Autodesk Inventor part; units mm, degrees
(part 2 of 3)
  spline S187 degree 2 poles (-30.3145, -0.1752) (-30.3145, 0.4002) (-30.6954, 1.2146) (-31.0722, 1.4456) knots 0 0 0 1 2 2 2
  spline S188 degree 2 poles (-31.0722, 1.4456) (-31.3396, 1.6036) (-31.9433, 1.7454) (-32.3931, 1.7454) knots 0 0 0 1 2 2 2
  line L488 (-32.3931, 1.7454) -> (-32.8996, 1.7454)
  line L489 (-32.8996, 1.7454) -> (-32.8996, -2.1038)
  line L490 (-32.8996, -2.1038) -> (-32.3931, -2.1038)
  spline S189 degree 2 poles (-32.3931, -2.1038) (-31.9514, -2.1038) (-31.2829, -1.962) (-31.0114, -1.7716) knots 0 0 0 1 2 2 2
  spline S190 degree 2 poles (-31.0114, -1.7716) (-30.6629, -1.5366) (-30.3145, -0.7586) (-30.3145, -0.1752) knots 0 0 0 1 2 2 2
  line L491 (-23.1062, -2.6792) -> (-23.9693, -2.6792)
  line L492 (-23.9693, -2.6792) -> (-25.7967, -0.3534)
  line L493 (-25.7967, -0.3534) -> (-26.0884, -0.6816)
  line L494 (-26.0884, -0.6816) -> (-26.0884, -2.6792)
  line L495 (-26.0884, -2.6792) -> (-26.7529, -2.6792)
  line L496 (-26.7529, -2.6792) -> (-26.7529, 2.3208)
  line L497 (-26.7529, 2.3208) -> (-26.0884, 2.3208)
  line L498 (-26.0884, 2.3208) -> (-26.0884, 0.0234)
  line L499 (-26.0884, 0.0234) -> (-24.0381, 2.3208)
  line L500 (-24.0381, 2.3208) -> (-23.2278, 2.3208)
  line L501 (-23.2278, 2.3208) -> (-25.2983, 0.0882)
  line L502 (-25.2983, 0.0882) -> (-23.1062, -2.6792)
  line L503 (-20.9668, -2.6792) -> (-22.9036, -2.6792)
  line L504 (-22.9036, -2.6792) -> (-22.9036, -2.1687)
  line L505 (-22.9036, -2.1687) -> (-22.2675, -2.1687)
  line L506 (-22.2675, -2.1687) -> (-22.2675, 1.8103)
  line L507 (-22.2675, 1.8103) -> (-22.9036, 1.8103)
  line L508 (-22.9036, 1.8103) -> (-22.9036, 2.3208)
  line L509 (-22.9036, 2.3208) -> (-20.9668, 2.3208)
  line L510 (-20.9668, 2.3208) -> (-20.9668, 1.8103)
  line L511 (-20.9668, 1.8103) -> (-21.603, 1.8103)
  line L512 (-21.603, 1.8103) -> (-21.603, -2.1687)
  line L513 (-21.603, -2.1687) -> (-20.9668, -2.1687)
  line L514 (-20.9668, -2.1687) -> (-20.9668, -2.6792)
  line L515 (-20.1443, -2.6792) -> (-20.1443, 2.3208)
  line L516 (-20.1443, 2.3208) -> (-17.0163, 2.3208)
  line L517 (-17.0163, 2.3208) -> (-17.0163, 1.7292)
  line L518 (-17.0163, 1.7292) -> (-19.4798, 1.7292)
  line L519 (-19.4798, 1.7292) -> (-19.4798, 0.3597)
  line L520 (-19.4798, 0.3597) -> (-17.1824, 0.3597)
  line L521 (-17.1824, 0.3597) -> (-17.1824, -0.2319)
  line L522 (-17.1824, -0.2319) -> (-19.4798, -0.2319)
  line L523 (-19.4798, -0.2319) -> (-19.4798, -2.0876)
  line L524 (-19.4798, -2.0876) -> (-17.0163, -2.0876)
  line L525 (-17.0163, -2.0876) -> (-17.0163, -2.6792)
  line L526 (-17.0163, -2.6792) -> (-20.1443, -2.6792)
  line L527 (-12.4174, -2.6792) -> (-13.2804, -2.6792)
  line L528 (-13.2804, -2.6792) -> (-14.8607, -0.6897)
  line L529 (-14.8607, -0.6897) -> (-15.6224, -0.6897)
  line L530 (-15.6224, -0.6897) -> (-15.6224, -2.6792)
  line L531 (-15.6224, -2.6792) -> (-16.2869, -2.6792)
  line L532 (-16.2869, -2.6792) -> (-16.2869, 2.3208)
  line L533 (-16.2869, 2.3208) -> (-14.9984, 2.3208)
  spline S191 degree 2 poles (-14.9984, 2.3208) (-14.5689, 2.3208) (-13.9895, 2.2276) (-13.7262, 2.0574) knots 0 0 0 1 2 2 2
  spline S192 degree 2 poles (-13.7262, 2.0574) (-13.4628, 1.8872) (-13.1589, 1.3564) (-13.1589, 0.9634) knots 0 0 0 1 2 2 2
  spline S193 degree 2 poles (-13.1589, 0.9634) (-13.1589, 0.4164) (-13.7181, -0.3251) (-14.1962, -0.5034) knots 0 0 0 1 2 2 2
  line L534 (-14.1962, -0.5034) -> (-12.4174, -2.6792)
  spline S194 degree 2 poles (-13.8518, 0.9107) (-13.8518, 1.1295) (-14.0057, 1.4658) (-14.1678, 1.5752) knots 0 0 0 1 2 2 2
  spline S195 degree 2 poles (-14.1678, 1.5752) (-14.3096, 1.6684) (-14.6864, 1.7454) (-14.962, 1.7454) knots 0 0 0 1 2 2 2
  line L535 (-14.962, 1.7454) -> (-15.6224, 1.7454)
  line L536 (-15.6224, 1.7454) -> (-15.6224, -0.1346)
  line L537 (-15.6224, -0.1346) -> (-15.039, -0.1346)
  spline S196 degree 2 poles (-15.039, -0.1346) (-14.7513, -0.1346) (-14.2934, -0.0333) (-14.1354, 0.1247) knots 0 0 0 1 2 2 2
  spline S197 degree 2 poles (-14.1354, 0.1247) (-13.9895, 0.2624) (-13.8518, 0.6514) (-13.8518, 0.9107) knots 0 0 0 1 2 2 2
  spline S198 degree 2 poles (-10.274, -2.7846) (-10.7156, -2.7846) (-11.372, -2.5536) (-11.603, -2.3226) knots 0 0 0 1 2 2 2
  spline S199 degree 2 poles (-11.603, -2.3226) (-11.8663, -2.0633) (-12.0811, -1.334) (-12.0811, -0.7991) knots 0 0 0 1 2 2 2
  line L538 (-12.0811, -0.7991) -> (-12.0811, 2.3208)
  line L539 (-12.0811, 2.3208) -> (-11.4166, 2.3208)
  line L540 (-11.4166, 2.3208) -> (-11.4166, -0.7991)
  spline S200 degree 2 poles (-11.4166, -0.7991) (-11.4166, -1.1476) (-11.3275, -1.6176) (-11.2018, -1.8081) knots 0 0 0 1 2 2 2
  spline S201 degree 2 poles (-11.2018, -1.8081) (-11.0681, -2.0107) (-10.6062, -2.2173) (-10.274, -2.2173) knots 0 0 0 1 2 2 2
  spline S202 degree 2 poles (-10.274, -2.2173) (-9.962, -2.2173) (-9.4757, -2.0107) (-9.342, -1.8081) knots 0 0 0 1 2 2 2
  spline S203 degree 2 poles (-9.342, -1.8081) (-9.2164, -1.6176) (-9.1273, -1.1517) (-9.1273, -0.8154) knots 0 0 0 1 2 2 2
  line L541 (-9.1273, -0.8154) -> (-9.1273, 2.3208)
  line L542 (-9.1273, 2.3208) -> (-8.4628, 2.3208)
  line L543 (-8.4628, 2.3208) -> (-8.4628, -0.7991)
  spline S204 degree 2 poles (-8.4628, -0.7991) (-8.4628, -1.3218) (-8.6735, -2.0674) (-8.9409, -2.3226) knots 0 0 0 1 2 2 2
  spline S205 degree 2 poles (-8.9409, -2.3226) (-9.18, -2.5577) (-9.8121, -2.7846) (-10.274, -2.7846) knots 0 0 0 1 2 2 2
  line L544 (-3.9328, -2.6792) -> (-4.6783, -2.6792)
  line L545 (-4.6783, -2.6792) -> (-6.8907, 1.632)
  line L546 (-6.8907, 1.632) -> (-6.8907, -2.6792)
  line L547 (-6.8907, -2.6792) -> (-7.5106, -2.6792)
  line L548 (-7.5106, -2.6792) -> (-7.5106, 2.3208)
  line L549 (-7.5106, 2.3208) -> (-6.5665, 2.3208)
  line L550 (-6.5665, 2.3208) -> (-4.5527, -1.6379)
  line L551 (-4.5527, -1.6379) -> (-4.5527, 2.3208)
  line L552 (-4.5527, 2.3208) -> (-3.9328, 2.3208)
  line L553 (-3.9328, 2.3208) -> (-3.9328, -2.6792)
  line L554 (0.7268, -2.6792) -> (-0.1362, -2.6792)
  line L555 (-0.1362, -2.6792) -> (-1.9636, -0.3534)
  line L556 (-1.9636, -0.3534) -> (-2.2553, -0.6816)
  line L557 (-2.2553, -0.6816) -> (-2.2553, -2.6792)
  line L558 (-2.2553, -2.6792) -> (-2.9198, -2.6792)
  line L559 (-2.9198, -2.6792) -> (-2.9198, 2.3208)
  line L560 (-2.9198, 2.3208) -> (-2.2553, 2.3208)
  line L561 (-2.2553, 2.3208) -> (-2.2553, 0.0234)
  line L562 (-2.2553, 0.0234) -> (-0.2051, 2.3208)
  line L563 (-0.2051, 2.3208) -> (0.6053, 2.3208)
  line L564 (0.6053, 2.3208) -> (-1.4652, 0.0882)
  line L565 (-1.4652, 0.0882) -> (0.7268, -2.6792)
  line L566 (2.8662, -2.6792) -> (0.9294, -2.6792)
  line L567 (0.9294, -2.6792) -> (0.9294, -2.1687)
  line L568 (0.9294, -2.1687) -> (1.5656, -2.1687)
  line L569 (1.5656, -2.1687) -> (1.5656, 1.8103)
  line L570 (1.5656, 1.8103) -> (0.9294, 1.8103)
  line L571 (0.9294, 1.8103) -> (0.9294, 2.3208)
  line L572 (0.9294, 2.3208) -> (2.8662, 2.3208)
  line L573 (2.8662, 2.3208) -> (2.8662, 1.8103)
  line L574 (2.8662, 1.8103) -> (2.2301, 1.8103)
  line L575 (2.2301, 1.8103) -> (2.2301, -2.1687)
  line L576 (2.2301, -2.1687) -> (2.8662, -2.1687)
  line L577 (2.8662, -2.1687) -> (2.8662, -2.6792)
  line L578 (3.6888, -2.6792) -> (3.6888, 2.3208)
  line L579 (3.6888, 2.3208) -> (6.8168, 2.3208)
  line L580 (6.8168, 2.3208) -> (6.8168, 1.7292)
  line L581 (6.8168, 1.7292) -> (4.3533, 1.7292)
  line L582 (4.3533, 1.7292) -> (4.3533, 0.3597)
  line L583 (4.3533, 0.3597) -> (6.6507, 0.3597)
  line L584 (6.6507, 0.3597) -> (6.6507, -0.2319)
  line L585 (6.6507, -0.2319) -> (4.3533, -0.2319)
  line L586 (4.3533, -0.2319) -> (4.3533, -2.0876)
  line L587 (4.3533, -2.0876) -> (6.8168, -2.0876)
  line L588 (6.8168, -2.0876) -> (6.8168, -2.6792)
  line L589 (6.8168, -2.6792) -> (3.6888, -2.6792)
  line L590 (11.833, -2.6792) -> (11.1685, -2.6792)
  line L591 (11.1685, -2.6792) -> (11.1685, 1.6279)
  line L592 (11.1685, 1.6279) -> (9.8638, -1.3016)
  line L593 (9.8638, -1.3016) -> (9.4586, -1.3016)
  line L594 (9.4586, -1.3016) -> (8.1661, 1.6279)
  line L595 (8.1661, 1.6279) -> (8.1661, -2.6792)
  line L596 (8.1661, -2.6792) -> (7.5461, -2.6792)
  line L597 (7.5461, -2.6792) -> (7.5461, 2.3208)
  line L598 (7.5461, 2.3208) -> (8.4537, 2.3208)
  line L599 (8.4537, 2.3208) -> (9.7017, -0.4628)
  line L600 (9.7017, -0.4628) -> (10.9092, 2.3208)
  line L601 (10.9092, 2.3208) -> (11.833, 2.3208)
  line L602 (11.833, 2.3208) -> (11.833, -2.6792)
  line L603 (16.7358, -2.6792) -> (14.799, -2.6792)
  line L604 (14.799, -2.6792) -> (14.799, -2.1687)
  line L605 (14.799, -2.1687) -> (15.4351, -2.1687)
  line L606 (15.4351, -2.1687) -> (15.4351, 1.8103)
  line L607 (15.4351, 1.8103) -> (14.799, 1.8103)
  line L608 (14.799, 1.8103) -> (14.799, 2.3208)
  line L609 (14.799, 2.3208) -> (16.7358, 2.3208)
  line L610 (16.7358, 2.3208) -> (16.7358, 1.8103)
  line L611 (16.7358, 1.8103) -> (16.0996, 1.8103)
  line L612 (16.0996, 1.8103) -> (16.0996, -2.1687)
  line L613 (16.0996, -2.1687) -> (16.7358, -2.1687)
  line L614 (16.7358, -2.1687) -> (16.7358, -2.6792)
  spline S206 degree 2 poles (23.2431, 1.7495) (23.5267, 1.4172) (23.8427, 0.4448) (23.8427, -0.1792) knots 0 0 0 1 2 2 2
  spline S207 degree 2 poles (23.8427, -0.1792) (23.8427, -0.787) (23.5348, -1.7716) (23.2431, -2.1038) knots 0 0 0 1 2 2 2
  spline S208 degree 2 poles (23.2431, -2.1038) (22.9351, -2.4523) (22.1207, -2.7846) (21.6304, -2.7846) knots 0 0 0 1 2 2 2
  spline S209 degree 2 poles (21.6304, -2.7846) (21.1239, -2.7846) (20.3136, -2.4402) (20.0178, -2.1038) knots 0 0 0 1 2 2 2
  spline S210 degree 2 poles (20.0178, -2.1038) (19.7301, -1.7716) (19.4221, -0.7951) (19.4221, -0.1792) knots 0 0 0 1 2 2 2
  spline S211 degree 2 poles (19.4221, -0.1792) (19.4221, 0.4488) (19.7341, 1.4051) (20.0218, 1.7495) knots 0 0 0 1 2 2 2
  spline S212 degree 2 poles (20.0218, 1.7495) (20.3136, 2.0817) (21.128, 2.4261) (21.6304, 2.4261) knots 0 0 0 1 2 2 2
  spline S213 degree 2 poles (21.6304, 2.4261) (22.1409, 2.4261) (22.9594, 2.0696) (23.2431, 1.7495) knots 0 0 0 1 2 2 2
  spline S214 degree 2 poles (23.1499, -0.1792) (23.1499, 0.3151) (22.9351, 1.0809) (22.7406, 1.3321) knots 0 0 0 1 2 2 2
  spline S215 degree 2 poles (22.7406, 1.3321) (22.5421, 1.5915) (21.9829, 1.8508) (21.6345, 1.8508) knots 0 0 0 1 2 2 2
  spline S216 degree 2 poles (21.6345, 1.8508) (21.2738, 1.8508) (20.7309, 1.5996) (20.5243, 1.3321) knots 0 0 0 1 2 2 2
  spline S217 degree 2 poles (20.5243, 1.3321) (20.3257, 1.0769) (20.115, 0.307) (20.115, -0.1792) knots 0 0 0 1 2 2 2
  spline S218 degree 2 poles (20.115, -0.1792) (20.115, -1.1638) (20.9416, -2.2092) (21.6345, -2.2092) knots 0 0 0 1 2 2 2
  spline S219 degree 2 poles (21.6345, -2.2092) (22.3273, -2.2092) (23.1499, -1.1638) (23.1499, -0.1792) knots 0 0 0 1 2 2 2
  spline S220 degree 2 poles (27.7325, 0.8135) (27.7325, 0.4893) (27.5016, -0.0941) (27.2949, -0.2967) knots 0 0 0 1 2 2 2
  spline S221 degree 2 poles (27.2949, -0.2967) (27.0356, -0.552) (26.3346, -0.8154) (25.7998, -0.8154) knots 0 0 0 1 2 2 2
  line L615 (25.7998, -0.8154) -> (25.2366, -0.8154)
  line L616 (25.2366, -0.8154) -> (25.2366, -2.6792)
  line L617 (25.2366, -2.6792) -> (24.5721, -2.6792)
  line L618 (24.5721, -2.6792) -> (24.5721, 2.3208)
  line L619 (24.5721, 2.3208) -> (25.8281, 2.3208)
  spline S222 degree 2 poles (25.8281, 2.3208) (26.2738, 2.3208) (26.8978, 2.1749) (27.1369, 2.0088) knots 0 0 0 1 2 2 2
  spline S223 degree 2 poles (27.1369, 2.0088) (27.4165, 1.8184) (27.7325, 1.2308) (27.7325, 0.8135) knots 0 0 0 1 2 2 2
  spline S224 degree 2 poles (27.0396, 0.7932) (27.0396, 1.0526) (26.8614, 1.4334) (26.679, 1.555) knots 0 0 0 1 2 2 2
  spline S225 degree 2 poles (26.679, 1.555) (26.521, 1.6603) (26.0996, 1.7454) (25.7876, 1.7454) knots 0 0 0 1 2 2 2
  line L620 (25.7876, 1.7454) -> (25.2366, 1.7454)
  line L621 (25.2366, 1.7454) -> (25.2366, -0.2481)
  line L622 (25.2366, -0.2481) -> (25.6904, -0.2481)
  spline S226 degree 2 poles (25.6904, -0.2481) (26.0956, -0.2481) (26.5939, -0.1184) (26.756, 0.0517) knots 0 0 0 1 2 2 2
  spline S227 degree 2 poles (26.756, 0.0517) (26.9059, 0.2017) (27.0396, 0.5542) (27.0396, 0.7932) knots 0 0 0 1 2 2 2
  line L623 (30.1069, -2.6792) -> (28.1701, -2.6792)
  line L624 (28.1701, -2.6792) -> (28.1701, -2.1687)
  line L625 (28.1701, -2.1687) -> (28.8063, -2.1687)
  line L626 (28.8063, -2.1687) -> (28.8063, 1.8103)
  line L627 (28.8063, 1.8103) -> (28.1701, 1.8103)
  line L628 (28.1701, 1.8103) -> (28.1701, 2.3208)
  line L629 (28.1701, 2.3208) -> (30.1069, 2.3208)
  line L630 (30.1069, 2.3208) -> (30.1069, 1.8103)
  line L631 (30.1069, 1.8103) -> (29.4708, 1.8103)
  line L632 (29.4708, 1.8103) -> (29.4708, -2.1687)
  line L633 (29.4708, -2.1687) -> (30.1069, -2.1687)
  line L634 (30.1069, -2.1687) -> (30.1069, -2.6792)
  line L635 (30.9294, -2.6792) -> (30.9294, 2.3208)
  line L636 (30.9294, 2.3208) -> (34.0575, 2.3208)
  line L637 (34.0575, 2.3208) -> (34.0575, 1.7292)
  line L638 (34.0575, 1.7292) -> (31.5939, 1.7292)
  line L639 (31.5939, 1.7292) -> (31.5939, 0.3597)
  line L640 (31.5939, 0.3597) -> (33.8913, 0.3597)
  line L641 (33.8913, 0.3597) -> (33.8913, -0.2319)
  line L642 (33.8913, -0.2319) -> (31.5939, -0.2319)
  line L643 (31.5939, -0.2319) -> (31.5939, -2.0876)
  line L644 (31.5939, -2.0876) -> (34.0575, -2.0876)
  line L645 (34.0575, -2.0876) -> (34.0575, -2.6792)
  line L646 (34.0575, -2.6792) -> (30.9294, -2.6792)
  line L647 (38.4335, -2.6792) -> (37.5704, -2.6792)
  line L648 (37.5704, -2.6792) -> (35.7431, -0.3534)
  line L649 (35.7431, -0.3534) -> (35.4513, -0.6816)
  line L650 (35.4513, -0.6816) -> (35.4513, -2.6792)
  line L651 (35.4513, -2.6792) -> (34.7868, -2.6792)
  line L652 (34.7868, -2.6792) -> (34.7868, 2.3208)
  line L653 (34.7868, 2.3208) -> (35.4513, 2.3208)
  line L654 (35.4513, 2.3208) -> (35.4513, 0.0234)
  line L655 (35.4513, 0.0234) -> (37.5016, 2.3208)
  line L656 (37.5016, 2.3208) -> (38.3119, 2.3208)
  line L657 (38.3119, 2.3208) -> (36.2414, 0.0882)
  line L658 (36.2414, 0.0882) -> (38.4335, -2.6792)
  line L659 (38.2917, -2.6792) -> (39.9772, 2.3208)
  line L660 (39.9772, 2.3208) -> (40.7957, 2.3208)
  line L661 (40.7957, 2.3208) -> (42.4813, -2.6792)
  line L662 (42.4813, -2.6792) -> (41.7803, -2.6792)
  line L663 (41.7803, -2.6792) -> (41.3265, -1.2813)
  line L664 (41.3265, -1.2813) -> (39.4181, -1.2813)
  line L665 (39.4181, -1.2813) -> (38.9643, -2.6792)
  line L666 (38.9643, -2.6792) -> (38.2917, -2.6792)
  line L667 (41.1442, -0.7141) -> (40.3703, 1.6401)
  line L668 (40.3703, 1.6401) -> (39.6004, -0.7141)
  line L669 (39.6004, -0.7141) -> (41.1442, -0.7141)
  spline S228 degree 2 poles (42.3597, -2.6792) (42.2139, -2.8008) (41.9951, -3.1614) (41.9951, -3.3194) knots 0 0 0 1 2 2 2
  spline S229 degree 2 poles (41.9951, -3.3194) (41.9951, -3.4288) (42.1207, -3.5666) (42.2463, -3.5666) knots 0 0 0 1 2 2 2
  spline S230 degree 2 poles (42.2463, -3.5666) (42.3152, -3.5666) (42.4408, -3.5342) (42.4813, -3.5179) knots 0 0 0 1 2 2 2
  line L670 (42.4813, -3.5179) -> (42.5178, -3.5179)
  line L671 (42.5178, -3.5179) -> (42.5178, -3.988)
  spline S231 degree 2 poles (42.5178, -3.988) (42.4205, -4.0285) (42.2058, -4.065) (42.1166, -4.065) knots 0 0 0 1 2 2 2
  spline S232 degree 2 poles (42.1166, -4.065) (41.8168, -4.065) (41.4764, -3.753) (41.4764, -3.4734) knots 0 0 0 1 2 2 2
  spline S233 degree 2 poles (41.4764, -3.4734) (41.4764, -3.2546) (41.7114, -2.821) (41.8614, -2.6792) knots 0 0 0 1 2 2 2
  line L672 (41.8614, -2.6792) -> (42.3597, -2.6792)
  line L673 (-22.1054, -10.9116) -> (-22.7699, -10.9116)
  line L674 (-22.7699, -10.9116) -> (-22.7699, -6.6045)
  line L675 (-22.7699, -6.6045) -> (-24.0746, -9.5339)
  line L676 (-24.0746, -9.5339) -> (-24.4798, -9.5339)
  line L677 (-24.4798, -9.5339) -> (-25.7723, -6.6045)
  line L678 (-25.7723, -6.6045) -> (-25.7723, -10.9116)
  line L679 (-25.7723, -10.9116) -> (-26.3923, -10.9116)
  line L680 (-26.3923, -10.9116) -> (-26.3923, -5.9116)
  line L681 (-26.3923, -5.9116) -> (-25.4847, -5.9116)
  line L682 (-25.4847, -5.9116) -> (-24.2367, -8.6952)
  line L683 (-24.2367, -8.6952) -> (-23.0292, -5.9116)
  line L684 (-23.0292, -5.9116) -> (-22.1054, -5.9116)
  line L685 (-22.1054, -5.9116) -> (-22.1054, -10.9116)
  line L686 (-21.0924, -10.9116) -> (-21.0924, -5.9116)
  line L687 (-21.0924, -5.9116) -> (-17.9644, -5.9116)
  line L688 (-17.9644, -5.9116) -> (-17.9644, -6.5032)
  line L689 (-17.9644, -6.5032) -> (-20.4279, -6.5032)
  line L690 (-20.4279, -6.5032) -> (-20.4279, -7.8727)
  line L691 (-20.4279, -7.8727) -> (-18.1305, -7.8727)
  line L692 (-18.1305, -7.8727) -> (-18.1305, -8.4643)
  line L693 (-18.1305, -8.4643) -> (-20.4279, -8.4643)
  line L694 (-20.4279, -8.4643) -> (-20.4279, -10.32)
  line L695 (-20.4279, -10.32) -> (-17.9644, -10.32)
  line L696 (-17.9644, -10.32) -> (-17.9644, -10.9116)
  line L697 (-17.9644, -10.9116) -> (-21.0924, -10.9116)
  line L698 (-13.3655, -10.9116) -> (-14.2286, -10.9116)
  line L699 (-14.2286, -10.9116) -> (-15.8088, -8.9221)
  line L700 (-15.8088, -8.9221) -> (-16.5706, -8.9221)
  line L701 (-16.5706, -8.9221) -> (-16.5706, -10.9116)
  line L702 (-16.5706, -10.9116) -> (-17.2351, -10.9116)
  line L703 (-17.2351, -10.9116) -> (-17.2351, -5.9116)
  line L704 (-17.2351, -5.9116) -> (-15.9466, -5.9116)
  spline S234 degree 2 poles (-15.9466, -5.9116) (-15.5171, -5.9116) (-14.9377, -6.0048) (-14.6743, -6.175) knots 0 0 0 1 2 2 2
  spline S235 degree 2 poles (-14.6743, -6.175) (-14.4109, -6.3451) (-14.107, -6.8759) (-14.107, -7.269) knots 0 0 0 1 2 2 2
  spline S236 degree 2 poles (-14.107, -7.269) (-14.107, -7.816) (-14.6662, -8.5574) (-15.1443, -8.7357) knots 0 0 0 1 2 2 2
  line L705 (-15.1443, -8.7357) -> (-13.3655, -10.9116)
  spline S237 degree 2 poles (-14.7999, -7.3216) (-14.7999, -7.1028) (-14.9539, -6.7665) (-15.1159, -6.6571) knots 0 0 0 1 2 2 2
  spline S238 degree 2 poles (-15.1159, -6.6571) (-15.2578, -6.5639) (-15.6346, -6.4869) (-15.9101, -6.4869) knots 0 0 0 1 2 2 2
  line L706 (-15.9101, -6.4869) -> (-16.5706, -6.4869)
  line L707 (-16.5706, -6.4869) -> (-16.5706, -8.367)
  line L708 (-16.5706, -8.367) -> (-15.9871, -8.367)
  spline S239 degree 2 poles (-15.9871, -8.367) (-15.6994, -8.367) (-15.2416, -8.2657) (-15.0835, -8.1077) knots 0 0 0 1 2 2 2
  spline S240 degree 2 poles (-15.0835, -8.1077) (-14.9377, -7.9699) (-14.7999, -7.5809) (-14.7999, -7.3216) knots 0 0 0 1 2 2 2
  line L709 (-9.4676, -5.9116) -> (-11.1573, -8.6993)
  line L710 (-11.1573, -8.6993) -> (-11.1573, -10.9116)
  line L711 (-11.1573, -10.9116) -> (-11.8218, -10.9116)
  line L712 (-11.8218, -10.9116) -> (-11.8218, -8.7681)
  line L713 (-11.8218, -8.7681) -> (-13.5114, -5.9116)
  line L714 (-13.5114, -5.9116) -> (-12.774, -5.9116)
  line L715 (-12.774, -5.9116) -> (-11.4855, -8.1117)
  line L716 (-11.4855, -8.1117) -> (-10.1727, -5.9116)
  line L717 (-10.1727, -5.9116) -> (-9.4676, -5.9116)
  line L718 (-7.8388, -10.9116) -> (-7.8388, -6.5032)
  line L719 (-7.8388, -6.5032) -> (-9.5163, -6.5032)
  line L720 (-9.5163, -6.5032) -> (-9.5163, -5.9116)
  line L721 (-9.5163, -5.9116) -> (-5.4968, -5.9116)
  line L722 (-5.4968, -5.9116) -> (-5.4968, -6.5032)
  line L723 (-5.4968, -6.5032) -> (-7.1743, -6.5032)
  line L724 (-7.1743, -6.5032) -> (-7.1743, -10.9116)
  line L725 (-7.1743, -10.9116) -> (-7.8388, -10.9116)
  spline S241 degree 2 poles (-1.4531, -6.4829) (-1.1694, -6.8151) (-0.8534, -7.7876) (-0.8534, -8.4116) knots 0 0 0 1 2 2 2
  spline S242 degree 2 poles (-0.8534, -8.4116) (-0.8534, -9.0194) (-1.1613, -10.004) (-1.4531, -10.3362) knots 0 0 0 1 2 2 2
  spline S243 degree 2 poles (-1.4531, -10.3362) (-1.761, -10.6847) (-2.5754, -11.0169) (-3.0657, -11.0169) knots 0 0 0 1 2 2 2
  spline S244 degree 2 poles (-3.0657, -11.0169) (-3.5722, -11.0169) (-4.3826, -10.6725) (-4.6783, -10.3362) knots 0 0 0 1 2 2 2
  spline S245 degree 2 poles (-4.6783, -10.3362) (-4.966, -10.004) (-5.274, -9.0275) (-5.274, -8.4116) knots 0 0 0 1 2 2 2
  spline S246 degree 2 poles (-5.274, -8.4116) (-5.274, -7.7835) (-4.962, -6.8273) (-4.6743, -6.4829) knots 0 0 0 1 2 2 2
  spline S247 degree 2 poles (-4.6743, -6.4829) (-4.3826, -6.1506) (-3.5681, -5.8062) (-3.0657, -5.8062) knots 0 0 0 1 2 2 2
  spline S248 degree 2 poles (-3.0657, -5.8062) (-2.5552, -5.8062) (-1.7367, -6.1628) (-1.4531, -6.4829) knots 0 0 0 1 2 2 2
  spline S249 degree 2 poles (-1.5463, -8.4116) (-1.5463, -7.9173) (-1.761, -7.1515) (-1.9555, -6.9002) knots 0 0 0 1 2 2 2
  spline S250 degree 2 poles (-1.9555, -6.9002) (-2.154, -6.6409) (-2.7132, -6.3816) (-3.0616, -6.3816) knots 0 0 0 1 2 2 2
  spline S251 degree 2 poles (-3.0616, -6.3816) (-3.4223, -6.3816) (-3.9652, -6.6328) (-4.1719, -6.9002) knots 0 0 0 1 2 2 2
  spline S252 degree 2 poles (-4.1719, -6.9002) (-4.3704, -7.1555) (-4.5811, -7.9254) (-4.5811, -8.4116) knots 0 0 0 1 2 2 2
  spline S253 degree 2 poles (-4.5811, -8.4116) (-4.5811, -9.3962) (-3.7545, -10.4416) (-3.0616, -10.4416) knots 0 0 0 1 2 2 2
  spline S254 degree 2 poles (-3.0616, -10.4416) (-2.3688, -10.4416) (-1.5463, -9.3962) (-1.5463, -8.4116) knots 0 0 0 1 2 2 2
  line L726 (3.7455, -10.9116) -> (2.8824, -10.9116)
  line L727 (2.8824, -10.9116) -> (1.3022, -8.9221)
  line L728 (1.3022, -8.9221) -> (0.5405, -8.9221)
  line L729 (0.5405, -8.9221) -> (0.5405, -10.9116)
  line L730 (0.5405, -10.9116) -> (-0.124, -10.9116)
  line L731 (-0.124, -10.9116) -> (-0.124, -5.9116)
  line L732 (-0.124, -5.9116) -> (1.1644, -5.9116)
  spline S255 degree 2 poles (1.1644, -5.9116) (1.5939, -5.9116) (2.1734, -6.0048) (2.4367, -6.175) knots 0 0 0 1 2 2 2
  spline S256 degree 2 poles (2.4367, -6.175) (2.7001, -6.3451) (3.004, -6.8759) (3.004, -7.269) knots 0 0 0 1 2 2 2
  spline S257 degree 2 poles (3.004, -7.269) (3.004, -7.816) (2.4448, -8.5574) (1.9667, -8.7357) knots 0 0 0 1 2 2 2
  line L733 (1.9667, -8.7357) -> (3.7455, -10.9116)
  spline S258 degree 2 poles (2.3111, -7.3216) (2.3111, -7.1028) (2.1572, -6.7665) (1.9951, -6.6571) knots 0 0 0 1 2 2 2
  spline S259 degree 2 poles (1.9951, -6.6571) (1.8533, -6.5639) (1.4764, -6.4869) (1.2009, -6.4869) knots 0 0 0 1 2 2 2
  line L734 (1.2009, -6.4869) -> (0.5405, -6.4869)
  line L735 (0.5405, -6.4869) -> (0.5405, -8.367)
  line L736 (0.5405, -8.367) -> (1.1239, -8.367)
  spline S260 degree 2 poles (1.1239, -8.367) (1.4116, -8.367) (1.8695, -8.2657) (2.0275, -8.1077) knots 0 0 0 1 2 2 2
  spline S261 degree 2 poles (2.0275, -8.1077) (2.1734, -7.9699) (2.3111, -7.5809) (2.3111, -7.3216) knots 0 0 0 1 2 2 2
  line L737 (7.6434, -5.9116) -> (5.9537, -8.6993)
  line L738 (5.9537, -8.6993) -> (5.9537, -10.9116)
  line L739 (5.9537, -10.9116) -> (5.2892, -10.9116)
  line L740 (5.2892, -10.9116) -> (5.2892, -8.7681)
  line L741 (5.2892, -8.7681) -> (3.5996, -5.9116)
  line L742 (3.5996, -5.9116) -> (4.3371, -5.9116)
  line L743 (4.3371, -5.9116) -> (5.6255, -8.1117)
  line L744 (5.6255, -8.1117) -> (6.9384, -5.9116)
  line L745 (6.9384, -5.9116) -> (7.6434, -5.9116)
  spline S262 degree 2 poles (10.0583, -11.0007) (9.5721, -11.0007) (8.7495, -10.6725) (8.4497, -10.3443) knots 0 0 0 1 2 2 2
  spline S263 degree 2 poles (8.4497, -10.3443) (8.1499, -10.0202) (7.8217, -9.0477) (7.8217, -8.4156) knots 0 0 0 1 2 2 2
  spline S264 degree 2 poles (7.8217, -8.4156) (7.8217, -7.7876) (8.1418, -6.8557) (8.4456, -6.5113) knots 0 0 0 1 2 2 2
  spline S265 degree 2 poles (8.4456, -6.5113) (8.7455, -6.175) (9.564, -5.8224) (10.0704, -5.8224) knots 0 0 0 1 2 2 2
  spline S266 degree 2 poles (10.0704, -5.8224) (10.3217, -5.8224) (10.7633, -5.8954) (10.9497, -5.9521) knots 0 0 0 1 2 2 2
  spline S267 degree 2 poles (10.9497, -5.9521) (11.1118, -6.0048) (11.4481, -6.1547) (11.6142, -6.2438) knots 0 0 0 1 2 2 2
  line L746 (11.6142, -6.2438) -> (11.6142, -7.0461)
  line L747 (11.6142, -7.0461) -> (11.5615, -7.0461)
  spline S268 degree 2 poles (11.5615, -7.0461) (11.4724, -6.9651) (11.1969, -6.7382) (10.9983, -6.6288) knots 0 0 0 1 2 2 2
  spline S269 degree 2 poles (10.9983, -6.6288) (10.8079, -6.5234) (10.3581, -6.3897) (10.0664, -6.3897) knots 0 0 0 1 2 2 2
  spline S270 degree 2 poles (10.0664, -6.3897) (9.7463, -6.3897) (9.175, -6.6531) (8.9602, -6.9043) knots 0 0 0 1 2 2 2
  spline S271 degree 2 poles (8.9602, -6.9043) (8.7495, -7.1596) (8.5145, -7.9335) (8.5145, -8.4156) knots 0 0 0 1 2 2 2
  spline S272 degree 2 poles (8.5145, -8.4156) (8.5145, -8.9302) (8.7617, -9.6717) (8.9764, -9.927) knots 0 0 0 1 2 2 2
  spline S273 degree 2 poles (8.9764, -9.927) (9.1871, -10.1741) (9.7503, -10.4254) (10.0664, -10.4254) knots 0 0 0 1 2 2 2
  spline S274 degree 2 poles (10.0664, -10.4254) (10.3541, -10.4254) (10.8443, -10.2835) (11.0348, -10.1782) knots 0 0 0 1 2 2 2
  spline S275 degree 2 poles (11.0348, -10.1782) (11.2171, -10.0728) (11.4886, -9.854) (11.5656, -9.7771) knots 0 0 0 1 2 2 2
  line L748 (11.5656, -9.7771) -> (11.6142, -9.7771)
  line L749 (11.6142, -9.7771) -> (11.6142, -10.5712)
  spline S276 degree 2 poles (11.6142, -10.5712) (11.4481, -10.6482) (11.1563, -10.79) (10.9497, -10.8549) knots 0 0 0 1 2 2 2
  spline S277 degree 2 poles (10.9497, -10.8549) (10.7309, -10.9278) (10.3581, -11.0007) (10.0583, -11.0007) knots 0 0 0 1 2 2 2
  line L750 (15.423, -10.9116) -> (11.9302, -10.9116)
  line L751 (11.9302, -10.9116) -> (11.9302, -10.2916)
  line L752 (11.9302, -10.2916) -> (14.6045, -6.5032)
  line L753 (14.6045, -6.5032) -> (12.0518, -6.5032)
  line L754 (12.0518, -6.5032) -> (12.0518, -5.9116)
  line L755 (12.0518, -5.9116) -> (15.3541, -5.9116)
  line L756 (15.3541, -5.9116) -> (15.3541, -6.5113)
  line L757 (15.3541, -6.5113) -> (12.6515, -10.32)
  line L758 (12.6515, -10.32) -> (15.423, -10.32)
  line L759 (15.423, -10.32) -> (15.423, -10.9116)
  line L760 (19.6572, -10.9116) -> (18.9116, -10.9116)
  line L761 (18.9116, -10.9116) -> (16.6993, -6.6004)
  line L762 (16.6993, -6.6004) -> (16.6993, -10.9116)
  line L763 (16.6993, -10.9116) -> (16.0794, -10.9116)
  line L764 (16.0794, -10.9116) -> (16.0794, -5.9116)
  line L765 (16.0794, -5.9116) -> (17.0234, -5.9116)
  line L766 (17.0234, -5.9116) -> (19.0372, -9.8703)
  line L767 (19.0372, -9.8703) -> (19.0372, -5.9116)
  line L768 (19.0372, -5.9116) -> (19.6572, -5.9116)
  line L769 (19.6572, -5.9116) -> (19.6572, -10.9116)
  line L770 (20.1312, -10.9116) -> (21.8168, -5.9116)
  line L771 (21.8168, -5.9116) -> (22.6353, -5.9116)
  line L772 (22.6353, -5.9116) -> (24.3208, -10.9116)
  line L773 (24.3208, -10.9116) -> (23.6199, -10.9116)
  line L774 (23.6199, -10.9116) -> (23.1661, -9.5137)
  line L775 (23.1661, -9.5137) -> (21.2576, -9.5137)
  line L776 (21.2576, -9.5137) -> (20.8038, -10.9116)
  line L777 (20.8038, -10.9116) -> (20.1312, -10.9116)
  line L778 (22.9837, -8.9464) -> (22.2098, -6.5923)
  line L779 (22.2098, -6.5923) -> (21.44, -8.9464)
  line L780 (21.44, -8.9464) -> (22.9837, -8.9464)
  spline S278 degree 2 poles (24.1993, -10.9116) (24.0534, -11.0331) (23.8346, -11.3938) (23.8346, -11.5518) knots 0 0 0 1 2 2 2
  spline S279 degree 2 poles (23.8346, -11.5518) (23.8346, -11.6612) (23.9602, -11.7989) (24.0858, -11.7989) knots 0 0 0 1 2 2 2
  spline S280 degree 2 poles (24.0858, -11.7989) (24.1547, -11.7989) (24.2803, -11.7665) (24.3208, -11.7503) knots 0 0 0 1 2 2 2
  line L781 (24.3208, -11.7503) -> (24.3573, -11.7503)
  line L782 (24.3573, -11.7503) -> (24.3573, -12.2203)
  spline S281 degree 2 poles (24.3573, -12.2203) (24.2601, -12.2609) (24.0453, -12.2973) (23.9562, -12.2973) knots 0 0 0 1 2 2 2
  spline S282 degree 2 poles (23.9562, -12.2973) (23.6563, -12.2973) (23.316, -11.9853) (23.316, -11.7057) knots 0 0 0 1 2 2 2
  spline S283 degree 2 poles (23.316, -11.7057) (23.316, -11.4869) (23.551, -11.0534) (23.7009, -10.9116) knots 0 0 0 1 2 2 2
  line L783 (23.7009, -10.9116) -> (24.1993, -10.9116)
  line L784 (25.9051, -10.9116) -> (25.1029, -10.9116)
  line L785 (25.1029, -10.9116) -> (25.1029, -9.9553)
  line L786 (25.1029, -9.9553) -> (25.9051, -9.9553)
  line L787 (25.9051, -9.9553) -> (25.9051, -10.9116)
  line L788 (25.9051, -8.1158) -> (25.1029, -8.1158)
  line L789 (25.1029, -8.1158) -> (25.1029, -7.1596)
  line L790 (25.1029, -7.1596) -> (25.9051, -7.1596)
  line L791 (25.9051, -7.1596) -> (25.9051, -8.1158)
  spline S284 degree 2 poles (-25.8331, -16.648) (-25.8331, -17.3328) (-26.3882, -18.4349) (-26.8542, -18.7428) knots 0 0 0 1 2 2 2
  spline S285 degree 2 poles (-26.8542, -18.7428) (-27.2351, -18.9819) (-28.0171, -19.1439) (-28.6249, -19.1439) knots 0 0 0 1 2 2 2
  line L792 (-28.6249, -19.1439) -> (-29.7756, -19.1439)
  line L793 (-29.7756, -19.1439) -> (-29.7756, -14.1439)
  line L794 (-29.7756, -14.1439) -> (-28.637, -14.1439)
  spline S286 degree 2 poles (-28.637, -14.1439) (-27.932, -14.1439) (-27.1297, -14.3546) (-26.8461, -14.541) knots 0 0 0 1 2 2 2
  spline S287 degree 2 poles (-26.8461, -14.541) (-26.3639, -14.8611) (-25.8331, -15.9187) (-25.8331, -16.648) knots 0 0 0 1 2 2 2
  spline S288 degree 2 poles (-26.526, -16.6399) (-26.526, -16.0645) (-26.9069, -15.2501) (-27.2837, -15.0192) knots 0 0 0 1 2 2 2
  spline S289 degree 2 poles (-27.2837, -15.0192) (-27.5511, -14.8611) (-28.1548, -14.7193) (-28.6046, -14.7193) knots 0 0 0 1 2 2 2
  line L795 (-28.6046, -14.7193) -> (-29.1111, -14.7193)
  line L796 (-29.1111, -14.7193) -> (-29.1111, -18.5686)
  line L797 (-29.1111, -18.5686) -> (-28.6046, -18.5686)
  spline S290 degree 2 poles (-28.6046, -18.5686) (-28.1629, -18.5686) (-27.4944, -18.4268) (-27.2229, -18.2363) knots 0 0 0 1 2 2 2
  spline S291 degree 2 poles (-27.2229, -18.2363) (-26.8745, -18.0013) (-26.526, -17.2234) (-26.526, -16.6399) knots 0 0 0 1 2 2 2
  line L798 (-21.2424, -19.1439) -> (-22.1054, -19.1439)
  line L799 (-22.1054, -19.1439) -> (-23.6856, -17.1545)
  line L800 (-23.6856, -17.1545) -> (-24.4474, -17.1545)
  line L801 (-24.4474, -17.1545) -> (-24.4474, -19.1439)
  line L802 (-24.4474, -19.1439) -> (-25.1119, -19.1439)
  line L803 (-25.1119, -19.1439) -> (-25.1119, -14.1439)
  line L804 (-25.1119, -14.1439) -> (-23.8234, -14.1439)
  spline S292 degree 2 poles (-23.8234, -14.1439) (-23.3939, -14.1439) (-22.8145, -14.2371) (-22.5511, -14.4073) knots 0 0 0 1 2 2 2
  spline S293 degree 2 poles (-22.5511, -14.4073) (-22.2877, -14.5775) (-21.9839, -15.1083) (-21.9839, -15.5013) knots 0 0 0 1 2 2 2
  spline S294 degree 2 poles (-21.9839, -15.5013) (-21.9839, -16.0483) (-22.543, -16.7898) (-23.0211, -16.9681) knots 0 0 0 1 2 2 2
  line L805 (-23.0211, -16.9681) -> (-21.2424, -19.1439)
  spline S295 degree 2 poles (-22.6767, -15.554) (-22.6767, -15.3352) (-22.8307, -14.9989) (-22.9928, -14.8895) knots 0 0 0 1 2 2 2
  spline S296 degree 2 poles (-22.9928, -14.8895) (-23.1346, -14.7963) (-23.5114, -14.7193) (-23.7869, -14.7193) knots 0 0 0 1 2 2 2
  line L806 (-23.7869, -14.7193) -> (-24.4474, -14.7193)
  line L807 (-24.4474, -14.7193) -> (-24.4474, -16.5994)
  line L808 (-24.4474, -16.5994) -> (-23.8639, -16.5994)
  spline S297 degree 2 poles (-23.8639, -16.5994) (-23.5762, -16.5994) (-23.1184, -16.4981) (-22.9604, -16.3401) knots 0 0 0 1 2 2 2
  spline S298 degree 2 poles (-22.9604, -16.3401) (-22.8145, -16.2023) (-22.6767, -15.8133) (-22.6767, -15.554) knots 0 0 0 1 2 2 2
  line L809 (-19.9134, -19.1439) -> (-20.7156, -19.1439)
  line L810 (-20.7156, -19.1439) -> (-20.7156, -18.1877)
  line L811 (-20.7156, -18.1877) -> (-19.9134, -18.1877)
  line L812 (-19.9134, -18.1877) -> (-19.9134, -19.1439)
  line L813 (-14.8728, -19.1439) -> (-16.8096, -19.1439)
  line L814 (-16.8096, -19.1439) -> (-16.8096, -18.6334)
  line L815 (-16.8096, -18.6334) -> (-16.1735, -18.6334)
  line L816 (-16.1735, -18.6334) -> (-16.1735, -14.6545)
  line L817 (-16.1735, -14.6545) -> (-16.8096, -14.6545)
  line L818 (-16.8096, -14.6545) -> (-16.8096, -14.1439)
  line L819 (-16.8096, -14.1439) -> (-14.8728, -14.1439)
  line L820 (-14.8728, -14.1439) -> (-14.8728, -14.6545)
  line L821 (-14.8728, -14.6545) -> (-15.509, -14.6545)
  line L822 (-15.509, -14.6545) -> (-15.509, -18.6334)
  line L823 (-15.509, -18.6334) -> (-14.8728, -18.6334)
  line L824 (-14.8728, -18.6334) -> (-14.8728, -19.1439)
  line L825 (-10.4725, -19.1439) -> (-11.2181, -19.1439)
  line L826 (-11.2181, -19.1439) -> (-13.4304, -14.8328)
  line L827 (-13.4304, -14.8328) -> (-13.4304, -19.1439)
  line L828 (-13.4304, -19.1439) -> (-14.0503, -19.1439)
  line L829 (-14.0503, -19.1439) -> (-14.0503, -14.1439)
  line L830 (-14.0503, -14.1439) -> (-13.1062, -14.1439)
  line L831 (-13.1062, -14.1439) -> (-11.0924, -18.1026)
  line L832 (-11.0924, -18.1026) -> (-11.0924, -14.1439)
  line L833 (-11.0924, -14.1439) -> (-10.4725, -14.1439)
  line L834 (-10.4725, -14.1439) -> (-10.4725, -19.1439)
  line L835 (-6.2707, -19.1439) -> (-9.7634, -19.1439)
  line L836 (-9.7634, -19.1439) -> (-9.7634, -18.524)
  line L837 (-9.7634, -18.524) -> (-7.0892, -14.7355)
  line L838 (-7.0892, -14.7355) -> (-9.6419, -14.7355)
  line L839 (-9.6419, -14.7355) -> (-9.6419, -14.1439)
  line L840 (-9.6419, -14.1439) -> (-6.3396, -14.1439)
  line L841 (-6.3396, -14.1439) -> (-6.3396, -14.7436)
  line L842 (-6.3396, -14.7436) -> (-9.0422, -18.5524)
  line L843 (-9.0422, -18.5524) -> (-6.2707, -18.5524)
  line L844 (-6.2707, -18.5524) -> (-6.2707, -19.1439)
  line L845 (-7.6565, -13.5119) -> (-8.3736, -13.5119)
  line L846 (-8.3736, -13.5119) -> (-8.3736, -12.8555)
  line L847 (-8.3736, -12.8555) -> (-7.6565, -12.8555)
  line L848 (-7.6565, -12.8555) -> (-7.6565, -13.5119)
  line L849 (-4.6824, -19.1439) -> (-5.4847, -19.1439)
  line L850 (-5.4847, -19.1439) -> (-5.4847, -18.1877)
  line L851 (-5.4847, -18.1877) -> (-4.6824, -18.1877)
  line L852 (-4.6824, -18.1877) -> (-4.6824, -19.1439)
  spline S299 degree 2 poles (2.5583, -16.648) (2.5583, -17.3328) (2.0032, -18.4349) (1.5372, -18.7428) knots 0 0 0 1 2 2 2
  spline S300 degree 2 poles (1.5372, -18.7428) (1.1563, -18.9819) (0.3743, -19.1439) (-0.2334, -19.1439) knots 0 0 0 1 2 2 2
  line L853 (-0.2334, -19.1439) -> (-1.3842, -19.1439)
  line L854 (-1.3842, -19.1439) -> (-1.3842, -14.1439)
  line L855 (-1.3842, -14.1439) -> (-0.2456, -14.1439)
  spline S301 degree 2 poles (-0.2456, -14.1439) (0.4594, -14.1439) (1.2617, -14.3546) (1.5453, -14.541) knots 0 0 0 1 2 2 2
  spline S302 degree 2 poles (1.5453, -14.541) (2.0275, -14.8611) (2.5583, -15.9187) (2.5583, -16.648) knots 0 0 0 1 2 2 2
  spline S303 degree 2 poles (1.8654, -16.6399) (1.8654, -16.0645) (1.4845, -15.2501) (1.1077, -15.0192) knots 0 0 0 1 2 2 2
  spline S304 degree 2 poles (1.1077, -15.0192) (0.8403, -14.8611) (0.2366, -14.7193) (-0.2132, -14.7193) knots 0 0 0 1 2 2 2
  line L856 (-0.2132, -14.7193) -> (-0.7197, -14.7193)
  line L857 (-0.7197, -14.7193) -> (-0.7197, -18.5686)
  line L858 (-0.7197, -18.5686) -> (-0.2132, -18.5686)
  spline S305 degree 2 poles (-0.2132, -18.5686) (0.2285, -18.5686) (0.897, -18.4268) (1.1685, -18.2363) knots 0 0 0 1 2 2 2
  spline S306 degree 2 poles (1.1685, -18.2363) (1.517, -18.0013) (1.8654, -17.2234) (1.8654, -16.6399) knots 0 0 0 1 2 2 2
  line L859 (2.7406, -19.1439) -> (4.4262, -14.1439)
  line L860 (4.4262, -14.1439) -> (5.2447, -14.1439)
  line L861 (5.2447, -14.1439) -> (6.9302, -19.1439)
  line L862 (6.9302, -19.1439) -> (6.2293, -19.1439)
  line L863 (6.2293, -19.1439) -> (5.7755, -17.7461)
  line L864 (5.7755, -17.7461) -> (3.867, -17.7461)
  line L865 (3.867, -17.7461) -> (3.4132, -19.1439)
  line L866 (3.4132, -19.1439) -> (2.7406, -19.1439)
  line L867 (5.5931, -17.1788) -> (4.8192, -14.8247)
  line L868 (4.8192, -14.8247) -> (4.0494, -17.1788)
  line L869 (4.0494, -17.1788) -> (5.5931, -17.1788)
  line L870 (11.2738, -19.1439) -> (10.4108, -19.1439)
  line L871 (10.4108, -19.1439) -> (8.8306, -17.1545)
  line L872 (8.8306, -17.1545) -> (8.0688, -17.1545)
  line L873 (8.0688, -17.1545) -> (8.0688, -19.1439)
  line L874 (8.0688, -19.1439) -> (7.4043, -19.1439)
  line L875 (7.4043, -19.1439) -> (7.4043, -14.1439)
  line L876 (7.4043, -14.1439) -> (8.6928, -14.1439)
  spline S307 degree 2 poles (8.6928, -14.1439) (9.1223, -14.1439) (9.7017, -14.2371) (9.9651, -14.4073) knots 0 0 0 1 2 2 2
  spline S308 degree 2 poles (9.9651, -14.4073) (10.2285, -14.5775) (10.5324, -15.1083) (10.5324, -15.5013) knots 0 0 0 1 2 2 2
  spline S309 degree 2 poles (10.5324, -15.5013) (10.5324, -16.0483) (9.9732, -16.7898) (9.4951, -16.9681) knots 0 0 0 1 2 2 2
  line L877 (9.4951, -16.9681) -> (11.2738, -19.1439)
  spline S310 degree 2 poles (9.8395, -15.554) (9.8395, -15.3352) (9.6855, -14.9989) (9.5234, -14.8895) knots 0 0 0 1 2 2 2
  spline S311 degree 2 poles (9.5234, -14.8895) (9.3816, -14.7963) (9.0048, -14.7193) (8.7293, -14.7193) knots 0 0 0 1 2 2 2
  line L878 (8.7293, -14.7193) -> (8.0688, -14.7193)
  line L879 (8.0688, -14.7193) -> (8.0688, -16.5994)
  line L880 (8.0688, -16.5994) -> (8.6523, -16.5994)
  spline S312 degree 2 poles (8.6523, -16.5994) (8.94, -16.5994) (9.3978, -16.4981) (9.5559, -16.3401) knots 0 0 0 1 2 2 2
  spline S313 degree 2 poles (9.5559, -16.3401) (9.7017, -16.2023) (9.8395, -15.8133) (9.8395, -15.554) knots 0 0 0 1 2 2 2
  line L881 (13.4132, -19.1439) -> (11.4764, -19.1439)
  line L882 (11.4764, -19.1439) -> (11.4764, -18.6334)
  line L883 (11.4764, -18.6334) -> (12.1126, -18.6334)
  line L884 (12.1126, -18.6334) -> (12.1126, -14.6545)
  line L885 (12.1126, -14.6545) -> (11.4764, -14.6545)
  line L886 (11.4764, -14.6545) -> (11.4764, -14.1439)
  line L887 (11.4764, -14.1439) -> (13.4132, -14.1439)
  line L888 (13.4132, -14.1439) -> (13.4132, -14.6545)
  line L889 (13.4132, -14.6545) -> (12.7771, -14.6545)
  line L890 (12.7771, -14.6545) -> (12.7771, -18.6334)
  line L891 (12.7771, -18.6334) -> (13.4132, -18.6334)
  line L892 (13.4132, -18.6334) -> (13.4132, -19.1439)
  spline S314 degree 2 poles (15.9821, -19.2493) (15.5405, -19.2493) (14.8841, -19.0183) (14.6531, -18.7874) knots 0 0 0 1 2 2 2
  spline S315 degree 2 poles (14.6531, -18.7874) (14.3897, -18.5281) (14.175, -17.7987) (14.175, -17.2639) knots 0 0 0 1 2 2 2
  line L893 (14.175, -17.2639) -> (14.175, -14.1439)
  line L894 (14.175, -14.1439) -> (14.8395, -14.1439)
  line L895 (14.8395, -14.1439) -> (14.8395, -17.2639)
  spline S316 degree 2 poles (14.8395, -17.2639) (14.8395, -17.6123) (14.9286, -18.0824) (15.0542, -18.2728) knots 0 0 0 1 2 2 2
  spline S317 degree 2 poles (15.0542, -18.2728) (15.1879, -18.4754) (15.6499, -18.682) (15.9821, -18.682) knots 0 0 0 1 2 2 2
  spline S318 degree 2 poles (15.9821, -18.682) (16.2941, -18.682) (16.7803, -18.4754) (16.914, -18.2728) knots 0 0 0 1 2 2 2
  spline S319 degree 2 poles (16.914, -18.2728) (17.0396, -18.0824) (17.1288, -17.6164) (17.1288, -17.2801) knots 0 0 0 1 2 2 2
  line L896 (17.1288, -17.2801) -> (17.1288, -14.1439)
  line L897 (17.1288, -14.1439) -> (17.7933, -14.1439)
  line L898 (17.7933, -14.1439) -> (17.7933, -17.2639)
  spline S320 degree 2 poles (17.7933, -17.2639) (17.7933, -17.7866) (17.5826, -18.5321) (17.3152, -18.7874) knots 0 0 0 1 2 2 2
  spline S321 degree 2 poles (17.3152, -18.7874) (17.0761, -19.0224) (16.444, -19.2493) (15.9821, -19.2493) knots 0 0 0 1 2 2 2
  spline S322 degree 2 poles (20.1393, -19.2331) (19.5964, -19.2331) (18.8346, -19.0062) (18.4983, -18.8441) knots 0 0 0 1 2 2 2
  line L899 (18.4983, -18.8441) -> (18.4983, -18.0094)
  line L900 (18.4983, -18.0094) -> (18.5469, -18.0094)
  spline S323 degree 2 poles (18.5469, -18.0094) (18.8751, -18.3174) (19.7058, -18.6577) (20.0907, -18.6577) knots 0 0 0 1 2 2 2
  spline S324 degree 2 poles (20.0907, -18.6577) (20.6418, -18.6577) (21.205, -18.1999) (21.205, -17.823) knots 0 0 0 1 2 2 2
  spline S325 degree 2 poles (21.205, -17.823) (21.205, -17.5232) (20.9092, -17.1504) (20.5891, -17.0572) knots 0 0 0 1 2 2 2
  spline S326 degree 2 poles (20.5891, -17.0572) (20.3581, -16.9924) (19.9732, -16.9033) (19.6855, -16.8303) knots 0 0 0 1 2 2 2
  spline S327 degree 2 poles (19.6855, -16.8303) (19.4262, -16.7615) (19.017, -16.5548) (18.8589, -16.3887) knots 0 0 0 1 2 2 2
  spline S328 degree 2 poles (18.8589, -16.3887) (18.705, -16.2226) (18.5348, -15.7769) (18.5348, -15.4851) knots 0 0 0 1 2 2 2
  spline S329 degree 2 poles (18.5348, -15.4851) (18.5348, -14.8773) (19.4829, -14.0548) (20.2163, -14.0548) knots 0 0 0 1 2 2 2
  spline S330 degree 2 poles (20.2163, -14.0548) (20.6377, -14.0548) (21.3832, -14.2209) (21.7033, -14.379) knots 0 0 0 1 2 2 2
  line L901 (21.7033, -14.379) -> (21.7033, -15.1731)
  line L902 (21.7033, -15.1731) -> (21.6547, -15.1731)
  spline S331 degree 2 poles (21.6547, -15.1731) (21.4157, -14.9543) (20.6701, -14.6302) (20.2609, -14.6302) knots 0 0 0 1 2 2 2
  spline S332 degree 2 poles (20.2609, -14.6302) (19.799, -14.6302) (19.2277, -15.0637) (19.2277, -15.4162) knots 0 0 0 1 2 2 2
  spline S333 degree 2 poles (19.2277, -15.4162) (19.2277, -15.7323) (19.564, -16.1091) (19.88, -16.1942) knots 0 0 0 1 2 2 2
  spline S334 degree 2 poles (19.88, -16.1942) (20.0907, -16.2509) (20.7025, -16.3968) (20.9051, -16.4576) knots 0 0 0 1 2 2 2
  spline S335 degree 2 poles (20.9051, -16.4576) (21.4197, -16.6156) (21.8978, -17.2517) (21.8978, -17.7177) knots 0 0 0 1 2 2 2
  spline S336 degree 2 poles (21.8978, -17.7177) (21.8978, -18.0135) (21.6588, -18.5807) (21.444, -18.7793) knots 0 0 0 1 2 2 2
  spline S337 degree 2 poles (21.444, -18.7793) (21.205, -18.9981) (20.5972, -19.2331) (20.1393, -19.2331) knots 0 0 0 1 2 2 2
  line L903 (25.7633, -19.1439) -> (22.2706, -19.1439)
  line L904 (22.2706, -19.1439) -> (22.2706, -18.524)
  line L905 (22.2706, -18.524) -> (24.9448, -14.7355)
  line L906 (24.9448, -14.7355) -> (22.3922, -14.7355)
  line L907 (22.3922, -14.7355) -> (22.3922, -14.1439)
  line L908 (22.3922, -14.1439) -> (25.6944, -14.1439)
  line L909 (25.6944, -14.1439) -> (25.6944, -14.7436)
  line L910 (25.6944, -14.7436) -> (22.9918, -18.5524)
  line L911 (22.9918, -18.5524) -> (25.7633, -18.5524)
  line L912 (25.7633, -18.5524) -> (25.7633, -19.1439)
  line L913 (25.8808, -19.1439) -> (27.5664, -14.1439)
  line L914 (27.5664, -14.1439) -> (28.3849, -14.1439)
  line L915 (28.3849, -14.1439) -> (30.0704, -19.1439)
  line L916 (30.0704, -19.1439) -> (29.3695, -19.1439)
  line L917 (29.3695, -19.1439) -> (28.9157, -17.7461)
  line L918 (28.9157, -17.7461) -> (27.0072, -17.7461)
  line L919 (27.0072, -17.7461) -> (26.5534, -19.1439)
  line L920 (26.5534, -19.1439) -> (25.8808, -19.1439)
  line L921 (28.7333, -17.1788) -> (27.9594, -14.8247)
  line L922 (27.9594, -14.8247) -> (27.1896, -17.1788)
  line L923 (27.1896, -17.1788) -> (28.7333, -17.1788)
  line L924 (-21.7104, -27.3763) -> (-22.3749, -27.3763)
  line L925 (-22.3749, -27.3763) -> (-22.3749, -23.0692)
  line L926 (-22.3749, -23.0692) -> (-23.6796, -25.9987)
  line L927 (-23.6796, -25.9987) -> (-24.0847, -25.9987)
  line L928 (-24.0847, -25.9987) -> (-25.3773, -23.0692)
  line L929 (-25.3773, -23.0692) -> (-25.3773, -27.3763)
  line L930 (-25.3773, -27.3763) -> (-25.9972, -27.3763)
  line L931 (-25.9972, -27.3763) -> (-25.9972, -22.3763)
  line L932 (-25.9972, -22.3763) -> (-25.0896, -22.3763)
  line L933 (-25.0896, -22.3763) -> (-23.8416, -25.1599)
  line L934 (-23.8416, -25.1599) -> (-22.6342, -22.3763)
  line L935 (-22.6342, -22.3763) -> (-21.7104, -22.3763)
  line L936 (-21.7104, -22.3763) -> (-21.7104, -27.3763)
  spline S338 degree 2 poles (-17.1601, -22.9476) (-16.8765, -23.2799) (-16.5604, -24.2523) (-16.5604, -24.8763) knots 0 0 0 1 2 2 2
  spline S339 degree 2 poles (-16.5604, -24.8763) (-16.5604, -25.4841) (-16.8684, -26.4687) (-17.1601, -26.801) knots 0 0 0 1 2 2 2
  spline S340 degree 2 poles (-17.1601, -26.801) (-17.4681, -27.1494) (-18.2825, -27.4817) (-18.7728, -27.4817) knots 0 0 0 1 2 2 2
  spline S341 degree 2 poles (-18.7728, -27.4817) (-19.2792, -27.4817) (-20.0896, -27.1373) (-20.3854, -26.801) knots 0 0 0 1 2 2 2
  spline S342 degree 2 poles (-20.3854, -26.801) (-20.6731, -26.4687) (-20.981, -25.4922) (-20.981, -24.8763) knots 0 0 0 1 2 2 2
  spline S343 degree 2 poles (-20.981, -24.8763) (-20.981, -24.2483) (-20.669, -23.292) (-20.3813, -22.9476) knots 0 0 0 1 2 2 2
  spline S344 degree 2 poles (-20.3813, -22.9476) (-20.0896, -22.6154) (-19.2752, -22.271) (-18.7728, -22.271) knots 0 0 0 1 2 2 2
  spline S345 degree 2 poles (-18.7728, -22.271) (-18.2622, -22.271) (-17.4437, -22.6275) (-17.1601, -22.9476) knots 0 0 0 1 2 2 2
  spline S346 degree 2 poles (-17.2533, -24.8763) (-17.2533, -24.382) (-17.4681, -23.6162) (-17.6625, -23.365) knots 0 0 0 1 2 2 2
  spline S347 degree 2 poles (-17.6625, -23.365) (-17.8611, -23.1057) (-18.4202, -22.8463) (-18.7687, -22.8463) knots 0 0 0 1 2 2 2
  spline S348 degree 2 poles (-18.7687, -22.8463) (-19.1293, -22.8463) (-19.6723, -23.0975) (-19.8789, -23.365) knots 0 0 0 1 2 2 2
  spline S349 degree 2 poles (-19.8789, -23.365) (-20.0775, -23.6202) (-20.2881, -24.3901) (-20.2881, -24.8763) knots 0 0 0 1 2 2 2
  spline S350 degree 2 poles (-20.2881, -24.8763) (-20.2881, -25.8609) (-19.4616, -26.9063) (-18.7687, -26.9063) knots 0 0 0 1 2 2 2
  spline S351 degree 2 poles (-18.7687, -26.9063) (-18.0758, -26.9063) (-17.2533, -25.8609) (-17.2533, -24.8763) knots 0 0 0 1 2 2 2
  spline S352 degree 2 poles (-14.4373, -27.4655) (-14.9802, -27.4655) (-15.742, -27.2386) (-16.0783, -27.0765) knots 0 0 0 1 2 2 2
  line L937 (-16.0783, -27.0765) -> (-16.0783, -26.2418)
  line L938 (-16.0783, -26.2418) -> (-16.0296, -26.2418)
  spline S353 degree 2 poles (-16.0296, -26.2418) (-15.7014, -26.5497) (-14.8708, -26.8901) (-14.4859, -26.8901) knots 0 0 0 1 2 2 2
  spline S354 degree 2 poles (-14.4859, -26.8901) (-13.9348, -26.8901) (-13.3716, -26.4322) (-13.3716, -26.0554) knots 0 0 0 1 2 2 2
  spline S355 degree 2 poles (-13.3716, -26.0554) (-13.3716, -25.7556) (-13.6674, -25.3828) (-13.9875, -25.2896) knots 0 0 0 1 2 2 2
  spline S356 degree 2 poles (-13.9875, -25.2896) (-14.2185, -25.2248) (-14.6034, -25.1356) (-14.8911, -25.0627) knots 0 0 0 1 2 2 2
  spline S357 degree 2 poles (-14.8911, -25.0627) (-15.1504, -24.9938) (-15.5596, -24.7872) (-15.7176, -24.6211) knots 0 0 0 1 2 2 2
  spline S358 degree 2 poles (-15.7176, -24.6211) (-15.8716, -24.4549) (-16.0418, -24.0092) (-16.0418, -23.7175) knots 0 0 0 1 2 2 2
  spline S359 degree 2 poles (-16.0418, -23.7175) (-16.0418, -23.1097) (-15.0937, -22.2872) (-14.3603, -22.2872) knots 0 0 0 1 2 2 2
  spline S360 degree 2 poles (-14.3603, -22.2872) (-13.9389, -22.2872) (-13.1933, -22.4533) (-12.8732, -22.6113) knots 0 0 0 1 2 2 2
  line L939 (-12.8732, -22.6113) -> (-12.8732, -23.4055)
  line L940 (-12.8732, -23.4055) -> (-12.9219, -23.4055)
  spline S361 degree 2 poles (-12.9219, -23.4055) (-13.1609, -23.1867) (-13.9065, -22.8625) (-14.3157, -22.8625) knots 0 0 0 1 2 2 2
  spline S362 degree 2 poles (-14.3157, -22.8625) (-14.7776, -22.8625) (-15.3489, -23.2961) (-15.3489, -23.6486) knots 0 0 0 1 2 2 2
  spline S363 degree 2 poles (-15.3489, -23.6486) (-15.3489, -23.9646) (-15.0126, -24.3415) (-14.6966, -24.4266) knots 0 0 0 1 2 2 2
  spline S364 degree 2 poles (-14.6966, -24.4266) (-14.4859, -24.4833) (-13.874, -24.6292) (-13.6715, -24.6899) knots 0 0 0 1 2 2 2
  spline S365 degree 2 poles (-13.6715, -24.6899) (-13.1569, -24.848) (-12.6787, -25.4841) (-12.6787, -25.9501) knots 0 0 0 1 2 2 2
  spline S366 degree 2 poles (-12.6787, -25.9501) (-12.6787, -26.2458) (-12.9178, -26.8131) (-13.1326, -27.0117) knots 0 0 0 1 2 2 2
  spline S367 degree 2 poles (-13.1326, -27.0117) (-13.3716, -27.2305) (-13.9794, -27.4655) (-14.4373, -27.4655) knots 0 0 0 1 2 2 2
  line L941 (-10.8352, -27.3763) -> (-10.8352, -22.9679)
  line L942 (-10.8352, -22.9679) -> (-12.5126, -22.9679)
  line L943 (-12.5126, -22.9679) -> (-12.5126, -22.3763)
  line L944 (-12.5126, -22.3763) -> (-8.4932, -22.3763)
  line L945 (-8.4932, -22.3763) -> (-8.4932, -22.9679)
  line L946 (-8.4932, -22.9679) -> (-10.1706, -22.9679)
  line L947 (-10.1706, -22.9679) -> (-10.1706, -27.3763)
  line L948 (-10.1706, -27.3763) -> (-10.8352, -27.3763)
  spline S368 degree 2 poles (-4.4494, -22.9476) (-4.1658, -23.2799) (-3.8497, -24.2523) (-3.8497, -24.8763) knots 0 0 0 1 2 2 2
  spline S369 degree 2 poles (-3.8497, -24.8763) (-3.8497, -25.4841) (-4.1577, -26.4687) (-4.4494, -26.801) knots 0 0 0 1 2 2 2
  spline S370 degree 2 poles (-4.4494, -26.801) (-4.7574, -27.1494) (-5.5718, -27.4817) (-6.0621, -27.4817) knots 0 0 0 1 2 2 2
  spline S371 degree 2 poles (-6.0621, -27.4817) (-6.5685, -27.4817) (-7.3789, -27.1373) (-7.6747, -26.801) knots 0 0 0 1 2 2 2
  spline S372 degree 2 poles (-7.6747, -26.801) (-7.9624, -26.4687) (-8.2703, -25.4922) (-8.2703, -24.8763) knots 0 0 0 1 2 2 2
  spline S373 degree 2 poles (-8.2703, -24.8763) (-8.2703, -24.2483) (-7.9583, -23.292) (-7.6706, -22.9476) knots 0 0 0 1 2 2 2
  spline S374 degree 2 poles (-7.6706, -22.9476) (-7.3789, -22.6154) (-6.5645, -22.271) (-6.0621, -22.271) knots 0 0 0 1 2 2 2
  spline S375 degree 2 poles (-6.0621, -22.271) (-5.5515, -22.271) (-4.733, -22.6275) (-4.4494, -22.9476) knots 0 0 0 1 2 2 2
  spline S376 degree 2 poles (-4.5426, -24.8763) (-4.5426, -24.382) (-4.7574, -23.6162) (-4.9518, -23.365) knots 0 0 0 1 2 2 2
  spline S377 degree 2 poles (-4.9518, -23.365) (-5.1504, -23.1057) (-5.7095, -22.8463) (-6.058, -22.8463) knots 0 0 0 1 2 2 2
  spline S378 degree 2 poles (-6.058, -22.8463) (-6.4186, -22.8463) (-6.9616, -23.0975) (-7.1682, -23.365) knots 0 0 0 1 2 2 2
  spline S379 degree 2 poles (-7.1682, -23.365) (-7.3668, -23.6202) (-7.5775, -24.3901) (-7.5775, -24.8763) knots 0 0 0 1 2 2 2
  spline S380 degree 2 poles (-7.5775, -24.8763) (-7.5775, -25.8609) (-6.7509, -26.9063) (-6.058, -26.9063) knots 0 0 0 1 2 2 2
  spline S381 degree 2 poles (-6.058, -26.9063) (-5.3651, -26.9063) (-4.5426, -25.8609) (-4.5426, -24.8763) knots 0 0 0 1 2 2 2
  line L949 (2.4833, -22.3763) -> (1.2272, -27.3763)
  line L950 (1.2272, -27.3763) -> (0.4817, -27.3763)
  line L951 (0.4817, -27.3763) -> (-0.5353, -23.2272)
  line L952 (-0.5353, -23.2272) -> (-1.524, -27.3763)
  line L953 (-1.524, -27.3763) -> (-2.2614, -27.3763)
  line L954 (-2.2614, -27.3763) -> (-3.5377, -22.3763)
  line L955 (-3.5377, -22.3763) -> (-2.853, -22.3763)